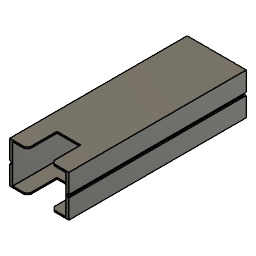
CASE_BATERIA (Autodesk Fusion 360 design; units mm, degrees)
Autodesk Fusion 360 part; units mm, degrees
sketch "Esboço1" plane through (0, 0, 0) normal (0, 1, 0) x (1, 0, 0)
  line L0 (0, 0) -> (20, 0)
  line L1 (0, 0) -> (-20, 0)
  line L2 (-20, 0) -> (-20, 120)
  line L3 (-20, 120) -> (20, 120)
  line L4 (20, 120) -> (20, 0)
  dimension "d1" = 20
  dimension "d2" = 20
  dimension "d3" = 120
  dimension "d4" = 40
  constraint coincident L0.start L1.start
  constraint horizontal L0
  constraint parallel L0 L1
  constraint perpendicular L1 L2
  constraint perpendicular L2 L3
  measures "d1" distance of L0.start L0.end
  measures "d2" distance of L0.start L1.end
  measures "d3" distance of L1.end L2.end
  measures "d4" distance of L2.end L3.end
extrude "Extrusão1" add sketch "Esboço1" along normal blind 28
sketch "Esboço2" plane through (0, 0, 0) normal (0, 0, 1) x (1, 0, 0)
  line L0 (-20, 0) -> (20, 0)
  line L1 (20, 0) -> (20, 28)
  line L2 (20, 28) -> (-20, 28)
  line L3 (-20, 28) -> (-20, 0)
  line L4 (0, 0) -> (0, 28) construction
  line L5 (0, 14) -> (0, 27)
  line L6 (0, 27) -> (18, 27)
  line L7 (18, 14) -> (18, 27)
  line L8 (18, 14) -> (18, 1)
  line L9 (18, 1) -> (0, 1)
  line L10 (-18, 1) -> (0, 1)
  line L11 (-18, 14) -> (-18, 1)
  line L12 (-18, 14) -> (-18, 27)
  line L13 (0, 27) -> (-18, 27)
  dimension "d7" = 18
  dimension "d9" = 13
  constraint coincident L4.start origin
  constraint midpoint L2 L4.end
  constraint midpoint L4 L5.start
  constraint perpendicular L1 L6
  constraint perpendicular L0 L8
  constraint coincident L4 L9.end
  constraint perpendicular L4 L9
  constraint symmetric L4 L7.start L11.start
  constraint symmetric L4 L5.end L6.start
  constraint symmetric L4 L6.end L12.end
  constraint symmetric L4 L8.end L10.start
  constraint symmetric L4 L9.end L10.end
  measures "d7" distance of L5.start L7.start
  measures "d9" distance of L5.start L5.end
extrude "Extrusão2" cut sketch "Esboço2" against normal blind 115 contours L6 L7 L8 L9 L10 L11 L12 L13
sketch "Esboço3" plane through (0, 28, 0) normal (0, 1, 0) x (-1, 0, 0)
  line L0 (20, 0) -> (-20, 0)
  line L1 (-20, 0) -> (-20, -120)
  line L2 (-20, -120) -> (20, -120)
  line L3 (20, -120) -> (20, 0)
  line L4 (0, 0) -> (10, 0)
  line L5 (0, 0) -> (-10, 0)
  line L6 (-8, -20) -> (8, -20)
  line L7 (-8, -2) -> (-8, -20)
  line L8 (8, -2) -> (8, -20)
  line L9 (10, 0) -> (7.8787, -2.1213)
  line L10 (-10, 0) -> (-7.8787, -2.1213)
  dimension "d13" = 10
  dimension "d14" = 10
  dimension "d19" = 135
  dimension "d20" = 3
  dimension "d22" = 3
  constraint coincident L4.start L5.start
  constraint parallel L0 L4
  constraint parallel L0 L5
  constraint perpendicular L6 L7
  constraint perpendicular L6 L8
  constraint coincident L9 L8.start
  constraint coincident L10 L7.start
  measures "d13" distance of L4.start L4.end
  measures "d14" distance of L4.start L5.end
  measures "d19" angle of L8 L9
  measures "d20" distance of L4.end L9.end
  measures "d22" distance of L5.end L10.end
extrude "Extrusão3" cut sketch "Esboço3" against normal blind 40 contours L0 L4 L5 L6 L7 L8 L9 L10
sketch "Esboço4" plane through (20, 0, 0) normal (1, 0, 0) x (0, 0, -1)
  line L0 (0, 0) -> (120, 0)
  line L1 (120, 0) -> (120, 28)
  line L2 (120, 28) -> (0, 28)
  line L3 (0, 28) -> (0, 0)
  line L4 (120, 14) -> (120, 14.9)
  line L5 (120, 14) -> (120, 13.1)
  line L6 (120, 13.1) -> (0, 13.1)
  line L7 (120, 14.9) -> (0, 14.9)
  line L8 (0, 14.9) -> (0, 13.1)
  dimension "d25" = 0.9
  dimension "d26" = 0.9
  constraint midpoint L1 L4.start
  constraint vertical L4
  constraint coincident L3 L6.end
  constraint perpendicular L3 L6
  constraint coincident L3 L7.end
  constraint perpendicular L3 L7
  measures "d25" distance of L4.start L4.end
  measures "d26" distance of L4.start L5.end
extrude "Extrusão4" cut sketch "Esboço4" against normal blind 1 contours L1 L3 L4 L5 L6 L7 L8
sketch "Esboço5" plane through (-20, 0, 0) normal (-1, 0, 0) x (0, 0, 1)
  line L0 (-120, 0) -> (0, 0)
  line L1 (0, 0) -> (0, 28)
  line L2 (0, 28) -> (-120, 28)
  line L3 (-120, 28) -> (-120, 0)
  line L4 (0, 13.1) -> (0, 14.9)
  line L5 (0, 14.9) -> (-120, 14.9)
  line L6 (0, 13.1) -> (-120, 13.1)
  line L7 (-120, 13.1) -> (-120, 13.3204)
  line L8 (-120, 14.9) -> (-120, 13.1)
  line L9 (-120, 13.1) -> (-120, 14.9)
  dimension "d30" = 1.8
  constraint coincident L3 L5.end
  constraint perpendicular L3 L5
  constraint coincident L3 L6.end
  constraint perpendicular L3 L6
  constraint coincident L3 L7.end
  measures "d30" distance of L4.start L4.end
extrude "Extrusão5" cut sketch "Esboço5" against normal blind 1 contours L1 L3 L4 L5 L6 L7 L8 L9
sketch "Esboço6" plane through (0, 0, -120) normal (0, 0, -1) x (-1, 0, 0)
  line L0 (20, 13.1) -> (19, 13.1)
  line L1 (19, 13.1) -> (19, 14.9)
  line L2 (19, 14.9) -> (20, 14.9)
  line L3 (20, 14.9) -> (20, 28)
  line L4 (20, 28) -> (-20, 28)
  line L5 (-20, 28) -> (-20, 14.9)
  line L6 (-20, 14.9) -> (-19, 14.9)
  line L7 (-19, 14.9) -> (-19, 13.1)
  line L8 (-19, 13.1) -> (-20, 13.1)
  line L9 (-20, 13.1) -> (-20, 0)
  line L10 (-20, 0) -> (20, 0)
  line L11 (20, 0) -> (20, 13.1)
  line L12 (-19, 14.9) -> (19, 14.9)
  line L13 (19, 13.1) -> (-19, 13.1)
  constraint coincident L6.end L7.start
  constraint coincident L1.end L2.start
  constraint coincident L0.end L1.start
  constraint coincident L7.end L8.start
extrude "Extrusão6" cut sketch "Esboço6" against normal blind 1 contours L1 L7 L12 L13
equation "d9 = ( 26 / 2 ) * 1 mm"
